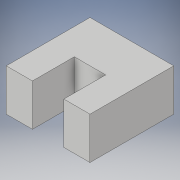
# Autodesk Inventor part: stand_holder
Saved by Autodesk Inventor 2019 (Build 230136000, 136)
## iProperties
Created: 2019-12-27
Part Number: stand_holder
Material: Типовые
Document SubType Name: Modeling
Designer: stepa
Density: 1 g/cm^3
Appearance: По умолчанию
Author: stepa
Autodesk Inventor part; units mm, degrees
ref_plane "YZ Plane" through (0, 0, 0) normal (1, 0, 0) x (0, 1, 0)
ref_plane "XZ Plane" through (0, 0, 0) normal (0, 1, 0) x (-1, 0, 0)
ref_plane "XY Plane" through (0, 0, 0) normal (0, 0, 1) x (1, 0, 0)
sketch "Эскиз1" plane through (0, 0, 0) normal (0, 1, 0) x (-1, 0, 0)
  line L0 (29.5774, -51.5004) -> (-50.4226, -51.5004)
  line L1 (-50.4226, -51.5004) -> (-50.4226, 28.4996)
  line L2 (-50.4226, 28.4996) -> (-25.4226, 28.4996)
  line L3 (-25.4226, 28.4996) -> (-25.4226, -11.5004)
  line L4 (-25.4226, -11.5004) -> (4.5774, -11.5004)
  line L5 (4.5774, -11.5004) -> (4.5774, 28.4996)
  line L6 (4.5774, 28.4996) -> (29.5774, 28.4996)
  line L7 (29.5774, 28.4996) -> (29.5774, -51.5004)
  point P0 (0, 0)
  dimension "d0" = 30
  dimension "d1" = 80
  dimension "d2" = 40
  dimension "d3" = 80
  constraints: 16 end point, 6 perpendicular, 2 point on line, 1 collinear, 1 horizontal
  measures "d0" distance of L3.end L4.end
  measures "d1" distance of L0.start L0.end
  measures "d2" distance between parallel lines of L0 L4
  measures "d3" distance of L6.end L0.start
extrude "Выдавливание1" add sketch "Эскиз1" along normal blind 40
